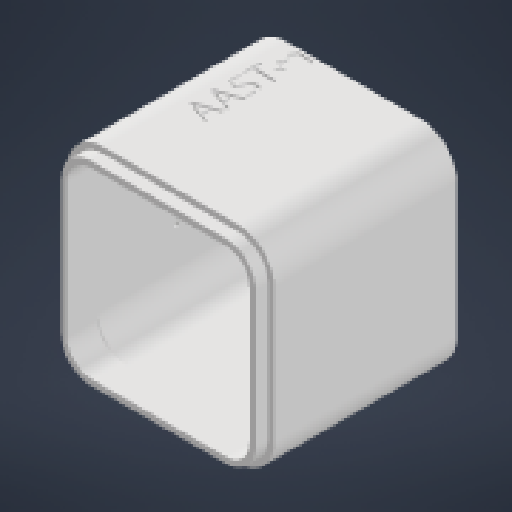
# Autodesk Inventor part: bottom case
Saved by Autodesk Inventor 2024 (Build 280153000, 153)
## iProperties
Created: 2023-06-18
Part Number: bottom case
Material: 일반
Document SubType Name: Modeling
Designer: 6gioc
Density: 1 g/cm^3
Appearance: 기본값
Author: 6gioc
Autodesk Inventor part; units mm, degrees
ref_plane "YZ Plane" through (0, 0, 0) normal (1, 0, 0) x (0, 1, 0)
ref_plane "XZ Plane" through (0, 0, 0) normal (0, 1, 0) x (-1, 0, 0)
ref_plane "XY Plane" through (0, 0, 0) normal (0, 0, 1) x (1, 0, 0)
sketch "스케치1" plane through (0, 0, 0) normal (0, 0, 1) x (1, 0, 0)
  line L0 (-30, 0) -> (-140, 0)
  line L1 (-170, -30) -> (-170, -140)
  line L2 (-140, -170) -> (-30, -170)
  line L3 (0, -140) -> (0, -30)
  arc A0 (-30, -170) -> (0, -140) centre (-30, -140) ccw
  arc A1 (-170, -140) -> (-140, -170) centre (-140, -140) ccw
  arc A2 (-140, 0) -> (-170, -30) centre (-140, -30) ccw
  arc A3 (0, -30) -> (-30, 0) centre (-30, -30) ccw
  point P0 (0, 0)
  point P1 (-170, -170)
  point P2 (-170, 0)
  point P3 (0, -170)
  dimension "d0" = 170
  dimension "d1" = 170
  dimension "d2" = 30
  dimension "d3" = 30
  dimension "d4" = 30
  constraints: 8 end point, 8 point on circle, 8 point on line, 8 tangent, 4 centre point, 2 parallel, 1 equal radius, 1 horizontal, 1 perpendicular
  measures "d0" distance of point (0, -170) point (-170, -170)
  measures "d1" distance of point (-170, -170) point (-170, 0)
  measures "d2" radius of A0
  measures "d3" radius of A1
  measures "d4" radius of A3
extrude "돌출1" add sketch "스케치1" along normal blind 150
shell "쉘1" thickness 5 removed faces 1 at (-66.6667, -113.3333, 150)
sketch "스케치2" plane through (0, 0, 150) normal (0, 0, 1) x (1, 0, 0)
  line L0 (-30, 0) -> (-140, 0)
  line L1 (-170, -30) -> (-170, -140)
  line L2 (-140, -170) -> (-30, -170)
  line L3 (0, -140) -> (0, -30)
  arc A0 (-30, -170) -> (0, -140) centre (-30, -140) ccw
  arc A1 (0, -30) -> (-30, 0) centre (-30, -30) ccw
  arc A2 (-140, 0) -> (-170, -30) centre (-140, -30) ccw
  arc A3 (-170, -140) -> (-140, -170) centre (-140, -140) ccw
  line L4 (-160, -30) -> (-160, -140)
  arc A4 (-160, -140) -> (-140, -160) centre (-140, -140) ccw
  line L5 (-140, -160) -> (-30, -160)
  arc A5 (-30, -160) -> (-10, -140) centre (-30, -140) ccw
  line L6 (-10, -140) -> (-10, -30)
  arc A6 (-10, -30) -> (-30, -10) centre (-30, -30) ccw
  line L7 (-30, -10) -> (-140, -10)
  arc A7 (-140, -10) -> (-160, -30) centre (-140, -30) ccw
  line L8 (-5, -140) -> (-5, -30)
  arc A8 (-5, -30) -> (-30, -5) centre (-30, -30) ccw
  line L9 (-30, -5) -> (-140, -5)
  arc A9 (-140, -5) -> (-165, -30) centre (-140, -30) ccw
  line L10 (-165, -30) -> (-165, -140)
  arc A10 (-165, -140) -> (-140, -165) centre (-140, -140) ccw
  line L11 (-140, -165) -> (-30, -165)
  arc A11 (-30, -165) -> (-5, -140) centre (-30, -140) ccw
  point P0 (0, 0)
  point P1 (-170, -170)
  point P2 (-170, 0)
  point P3 (0, -170)
  dimension "d8" = 170
  dimension "d9" = 170
  dimension "d10" = 30
  dimension "d11" = 10
  dimension "d17" = 5
  constraints: 24 end point, 24 point on circle, 12 centre point, 8 point on line, 8 tangent, 6 parallel, 3 equal radius, 3 perpendicular, 1 horizontal, 14 other
  measures "d8" distance of point (0, -170) point (-170, -170)
  measures "d9" distance of point (-170, -170) point (-170, 0)
  measures "d10" radius of A0
  measures "d11" radial gap between concentric circles of A2 A7
  measures "d17" radial gap between concentric circles of A0 A11
extrude "돌출2" add sketch "스케치2" against normal blind 20 contours A1 L3 A0 L2 A3 L1 A2 L0 | A11 L11 A10 L10 A9 L9 A8 L8
chamfer "모따기1" distance 5 angle 45 8 edges at (-85, -160, 130) (-15.8579, -154.1421, 130) (-10, -85, 130) (-15.8579, -15.8579, 130) (-85, -10, 130) (-154.1421, -15.8579, 130) (-160, -85, 130) (-154.1421, -154.1421, 130)
extrude "돌출3" add sketch "스케치2" along normal blind 10 contours A11 L11 A10 L10 A9 L9 A8 L8
sketch "스케치3" plane through (-140, 0, 0) normal (0, 1, 0) x (1, 0, 0)
  line L0 (23.785, -91.5699) -> (3.785, -84.2336)
  line L1 (3.785, -84.2336) -> (3.785, -81.9279)
  line L2 (3.785, -81.9279) -> (23.785, -74.6266)
  line L3 (23.785, -74.6266) -> (23.785, -77.107)
  line L4 (23.785, -77.107) -> (17.9509, -79.2205)
  line L5 (17.9509, -79.2205) -> (17.9509, -87.238)
  line L6 (17.9509, -87.238) -> (23.785, -89.2991)
  line L7 (23.785, -89.2991) -> (23.785, -91.5699)
  line L8 (6.9465, -83.2729) -> (15.9422, -86.5568)
  line L9 (15.9422, -86.5568) -> (15.9422, -79.9716)
  line L10 (15.9422, -79.9716) -> (6.9465, -83.2205)
  line L11 (6.9465, -83.2205) -> (6.9465, -83.2729)
  line L12 (23.785, -73.5262) -> (3.785, -66.1899)
  line L13 (3.785, -66.1899) -> (3.785, -63.8843)
  line L14 (3.785, -63.8843) -> (23.785, -56.583)
  line L15 (23.785, -56.583) -> (23.785, -59.0633)
  line L16 (23.785, -59.0633) -> (17.9509, -61.1768)
  line L17 (17.9509, -61.1768) -> (17.9509, -69.1943)
  line L18 (17.9509, -69.1943) -> (23.785, -71.2555)
  line L19 (23.785, -71.2555) -> (23.785, -73.5262)
  line L20 (6.9465, -65.2292) -> (15.9422, -68.5131)
  line L21 (15.9422, -68.5131) -> (15.9422, -61.9279)
  line L22 (15.9422, -61.9279) -> (6.9465, -65.1768)
  line L23 (6.9465, -65.1768) -> (6.9465, -65.2292)
  spline S0 degree 2 poles (24.1518, -49.1768) (24.1518, -52.4607) (22.8068, -54.8712) knots 0 0 0 1 1 1
  line L24 (22.8068, -54.8712) -> (20.8155, -54.8712)
  spline S1 degree 2 poles (20.8155, -54.8712) (22.1256, -52.321) (22.1256, -49.2817) knots 0 0 0 1 1 1
  spline S2 degree 2 poles (22.1256, -49.2817) (22.1256, -47.0284) (20.2042, -44.8624) (18.5098, -44.8624) knots 0 0 0 1 2 2 2
  spline S3 degree 2 poles (18.5098, -44.8624) (17.0251, -44.8624) (15.4356, -46.3821) (14.8417, -48.2511) knots 0 0 0 1 2 2 2
  line L25 (14.8417, -48.2511) -> (14.1605, -50.1899)
  spline S4 degree 2 poles (14.1605, -50.1899) (13.4094, -52.4083) (10.9465, -54.5742) (8.7631, -54.5742) knots 0 0 0 1 2 2 2
  spline S5 degree 2 poles (8.7631, -54.5742) (6.3526, -54.5742) (3.4531, -51.3952) (3.4531, -48.3559) knots 0 0 0 1 2 2 2
  spline S6 degree 2 poles (3.4531, -48.3559) (3.4531, -45.7533) (4.5535, -43.4825) knots 0 0 0 1 1 1
  line L26 (4.5535, -43.4825) -> (6.5622, -43.4825)
  spline S7 degree 2 poles (6.5622, -43.4825) (5.4443, -45.8755) (5.4443, -48.4432) knots 0 0 0 1 1 1
  spline S8 degree 2 poles (5.4443, -48.4432) (5.4443, -50.2598) (7.1212, -52.2511) (9.9858, -52.2511) (11.4705, -50.976) (12.0644, -49.2817) knots 0 0 0 1 2 3 4 4 4
  line L27 (12.0644, -49.2817) -> (12.6932, -47.3079)
  spline S9 degree 2 poles (12.6932, -47.3079) (13.5317, -44.8275) (15.9771, -42.4694) (18.3352, -42.4694) knots 0 0 0 1 2 2 2
  spline S10 degree 2 poles (18.3352, -42.4694) (21.0426, -42.4694) (24.1518, -45.7882) (24.1518, -49.1768) knots 0 0 0 1 2 2 2
  line L28 (23.785, -34.0677) -> (5.7762, -34.0677)
  line L29 (5.7762, -34.0677) -> (5.7762, -40.1812)
  line L30 (5.7762, -40.1812) -> (3.785, -40.1812)
  line L31 (3.785, -40.1812) -> (3.785, -25.631)
  line L32 (3.785, -25.631) -> (5.7762, -25.631)
  line L33 (5.7762, -25.631) -> (5.7762, -31.7445)
  line L34 (5.7762, -31.7445) -> (23.785, -31.7445)
  line L35 (23.785, -31.7445) -> (23.785, -34.0677)
  spline S11 degree 2 poles (9.9173, -17.3252) (11.1446, -16.9103) (12.5448, -14.4038) (12.5448, -13.1592) knots 0 0 0 1 2 2 2
  spline S12 degree 2 poles (12.5448, -13.1592) (12.5448, -11.6208) (10.9199, -8.9587) (9.416, -8.5438) knots 0 0 0 1 2 2 2
  spline S13 degree 2 poles (9.416, -8.5438) (9.8481, -6.7979) (11.8706, -3.7037) (12.804, -3.0469) knots 0 0 0 1 2 2 2
  spline S14 degree 2 poles (12.804, -3.0469) (13.8585, -2.3208) (15.2068, -2.3208) knots 0 0 0 1 1 1
  spline S15 degree 2 poles (15.2068, -2.3208) (16.123, -2.3208) (17.2811, -2.7703) knots 0 0 0 1 1 1
  spline S16 degree 2 poles (17.2811, -2.7703) (18.1973, -3.2197) (18.8369, -3.2197) knots 0 0 0 1 1 1
  spline S17 degree 2 poles (18.8369, -3.2197) (19.3036, -3.2197) (20.8594, -2.5801) knots 0 0 0 1 1 1
  spline S18 degree 2 poles (20.8594, -2.5801) (21.8447, -2.2863) (22.3114, -2.2863) knots 0 0 0 1 1 1
  spline S19 degree 2 poles (22.3114, -2.2863) (23.6943, -2.2863) (25.1117, -3.4617) knots 0 0 0 1 1 1
  spline S20 degree 2 poles (25.1117, -3.4617) (27.0651, -5.2422) (29.2258, -10.3243) (29.2258, -13.1074) knots 0 0 0 1 2 2 2
  spline S21 degree 2 poles (29.2258, -13.1074) (29.2258, -16.0114) (25.8378, -20.4367) (23.2103, -20.4367) knots 0 0 0 1 2 2 2
  spline S22 degree 2 poles (23.2103, -20.4367) (21.7755, -20.4367) (20.5482, -19.8144) knots 0 0 0 1 1 1
  spline S23 degree 2 poles (20.5482, -19.8144) (19.7185, -19.2958) (18.8715, -19.2958) knots 0 0 0 1 1 1
  spline S24 degree 2 poles (18.8715, -19.2958) (18.059, -19.2958) (17.2811, -19.6242) knots 0 0 0 1 1 1
  spline S25 degree 2 poles (17.2811, -19.6242) (15.2241, -20.4367) (14.4981, -20.4367) knots 0 0 0 1 1 1
  spline S26 degree 2 poles (14.4981, -20.4367) (12.5102, -20.4367) (11.0063, -19.0883) knots 0 0 0 1 1 1
  spline S27 degree 2 poles (11.0063, -19.0883) (10.384, -18.466) (9.9173, -17.3252) knots 0 0 0 1 1 1
  spline S28 degree 2 poles (19.7531, -19.6934) (19.7531, -21.8023) (18.3183, -23.5654) knots 0 0 0 1 1 1
  spline S29 degree 2 poles (18.3183, -23.5654) (16.97, -25.0348) (14.5672, -25.3805) knots 0 0 0 1 1 1
  spline S30 degree 2 poles (14.5672, -25.3805) (14.5672, -22.9604) (15.9328, -21.3528) knots 0 0 0 1 1 1
  spline S31 degree 2 poles (15.9328, -21.3528) (17.454, -19.6934) (19.7531, -19.6934) knots 0 0 0 1 1 1
  point P0 (140, 0)
  point P1 (3.4531, -92.1288)
  dimension "d0" = 170
  dimension "d1" = 170
  dimension "d2" = 30
  dimension "d3" = 30
  dimension "d4" = 30
  constraints: 1 other
extrude "돌출4" cut sketch "스케치3" against normal blind 2
sketch "스케치4" plane through (-140, -170, 0) normal (0, -1, 0) x (1, 0, 0)
  line L0 (-0.2518, 6.8609) -> (110.1783, 6.8609) construction
  line L1 (110.1783, 6.8609) -> (110.1783, 29.5331) construction
  line L2 (110.1783, 29.5331) -> (-0.2518, 29.5331) construction
  line L3 (-0.2518, 29.5331) -> (-0.2518, 6.8609) construction
  line L4 (6.2831, 27.3688) -> (5.0902, 27.3688)
  line L5 (5.0902, 27.3688) -> (1.5505, 34.2667)
  line L6 (1.5505, 34.2667) -> (1.5505, 27.3688)
  line L7 (1.5505, 27.3688) -> (0.5586, 27.3688)
  line L8 (0.5586, 27.3688) -> (0.5586, 35.3688)
  line L9 (0.5586, 35.3688) -> (2.0692, 35.3688)
  line L10 (2.0692, 35.3688) -> (5.2912, 29.0349)
  line L11 (5.2912, 29.0349) -> (5.2912, 35.3688)
  line L12 (5.2912, 35.3688) -> (6.2831, 35.3688)
  line L13 (6.2831, 35.3688) -> (6.2831, 27.3688)
  spline S0 degree 2 poles (13.5635, 34.4547) (14.0173, 33.9231) (14.523, 32.3672) (14.523, 31.3688) knots 0 0 0 1 2 2 2
  spline S1 degree 2 poles (14.523, 31.3688) (14.523, 30.3964) (14.0303, 28.821) (13.5635, 28.2894) knots 0 0 0 1 2 2 2
  spline S2 degree 2 poles (13.5635, 28.2894) (13.0708, 27.7319) (11.7677, 27.2002) (10.9833, 27.2002) knots 0 0 0 1 2 2 2
  spline S3 degree 2 poles (10.9833, 27.2002) (10.1729, 27.2002) (8.8763, 27.7513) (8.403, 28.2894) knots 0 0 0 1 2 2 2
  spline S4 degree 2 poles (8.403, 28.2894) (7.9427, 28.821) (7.45, 30.3834) (7.45, 31.3688) knots 0 0 0 1 2 2 2
  spline S5 degree 2 poles (7.45, 31.3688) (7.45, 32.3737) (7.9492, 33.9037) (8.4095, 34.4547) knots 0 0 0 1 2 2 2
  spline S6 degree 2 poles (8.4095, 34.4547) (8.8763, 34.9863) (10.1794, 35.5374) (10.9833, 35.5374) knots 0 0 0 1 2 2 2
  spline S7 degree 2 poles (10.9833, 35.5374) (11.8001, 35.5374) (13.1097, 34.9669) (13.5635, 34.4547) knots 0 0 0 1 2 2 2
  spline S8 degree 2 poles (13.4144, 31.3688) (13.4144, 32.1597) (13.0708, 33.385) (12.7596, 33.787) knots 0 0 0 1 2 2 2
  spline S9 degree 2 poles (12.7596, 33.787) (12.4419, 34.2019) (11.5473, 34.6168) (10.9897, 34.6168) knots 0 0 0 1 2 2 2
  spline S10 degree 2 poles (10.9897, 34.6168) (10.4128, 34.6168) (9.544, 34.2148) (9.2134, 33.787) knots 0 0 0 1 2 2 2
  spline S11 degree 2 poles (9.2134, 33.787) (8.8957, 33.3785) (8.5586, 32.1468) (8.5586, 31.3688) knots 0 0 0 1 2 2 2
  spline S12 degree 2 poles (8.5586, 31.3688) (8.5586, 29.7934) (9.8811, 28.1208) (10.9897, 28.1208) knots 0 0 0 1 2 2 2
  spline S13 degree 2 poles (10.9897, 28.1208) (12.0983, 28.1208) (13.4144, 29.7934) (13.4144, 31.3688) knots 0 0 0 1 2 2 2
  line L14 (17.557, 27.3688) -> (17.557, 34.4223)
  line L15 (17.557, 34.4223) -> (14.873, 34.4223)
  line L16 (14.873, 34.4223) -> (14.873, 35.3688)
  line L17 (14.873, 35.3688) -> (21.3042, 35.3688)
  line L18 (21.3042, 35.3688) -> (21.3042, 34.4223)
  line L19 (21.3042, 34.4223) -> (18.6202, 34.4223)
  line L20 (18.6202, 34.4223) -> (18.6202, 27.3688)
  line L21 (18.6202, 27.3688) -> (17.557, 27.3688)
  line L22 (30.335, 34.4223) -> (26.6137, 34.4223)
  line L23 (26.6137, 34.4223) -> (26.6137, 32.1662)
  line L24 (26.6137, 32.1662) -> (30.1794, 32.1662)
  line L25 (30.1794, 32.1662) -> (30.1794, 31.2197)
  line L26 (30.1794, 31.2197) -> (26.6137, 31.2197)
  line L27 (26.6137, 31.2197) -> (26.6137, 27.3688)
  line L28 (26.6137, 27.3688) -> (25.5505, 27.3688)
  line L29 (25.5505, 27.3688) -> (25.5505, 35.3688)
  line L30 (25.5505, 35.3688) -> (30.335, 35.3688)
  line L31 (30.335, 35.3688) -> (30.335, 34.4223)
  spline S14 degree 2 poles (36.9476, 34.4547) (37.4014, 33.9231) (37.9071, 32.3672) (37.9071, 31.3688) knots 0 0 0 1 2 2 2
  spline S15 degree 2 poles (37.9071, 31.3688) (37.9071, 30.3964) (37.4144, 28.821) (36.9476, 28.2894) knots 0 0 0 1 2 2 2
  spline S16 degree 2 poles (36.9476, 28.2894) (36.4549, 27.7319) (35.1518, 27.2002) (34.3674, 27.2002) knots 0 0 0 1 2 2 2
  spline S17 degree 2 poles (34.3674, 27.2002) (33.557, 27.2002) (32.2604, 27.7513) (31.7871, 28.2894) knots 0 0 0 1 2 2 2
  spline S18 degree 2 poles (31.7871, 28.2894) (31.3269, 28.821) (30.8341, 30.3834) (30.8341, 31.3688) knots 0 0 0 1 2 2 2
  spline S19 degree 2 poles (30.8341, 31.3688) (30.8341, 32.3737) (31.3333, 33.9037) (31.7936, 34.4547) knots 0 0 0 1 2 2 2
  spline S20 degree 2 poles (31.7936, 34.4547) (32.2604, 34.9863) (33.5635, 35.5374) (34.3674, 35.5374) knots 0 0 0 1 2 2 2
  spline S21 degree 2 poles (34.3674, 35.5374) (35.1842, 35.5374) (36.4938, 34.9669) (36.9476, 34.4547) knots 0 0 0 1 2 2 2
  spline S22 degree 2 poles (36.7985, 31.3688) (36.7985, 32.1597) (36.4549, 33.385) (36.1437, 33.787) knots 0 0 0 1 2 2 2
  spline S23 degree 2 poles (36.1437, 33.787) (35.826, 34.2019) (34.9314, 34.6168) (34.3739, 34.6168) knots 0 0 0 1 2 2 2
  spline S24 degree 2 poles (34.3739, 34.6168) (33.7969, 34.6168) (32.9281, 34.2148) (32.5975, 33.787) knots 0 0 0 1 2 2 2
  spline S25 degree 2 poles (32.5975, 33.787) (32.2799, 33.3785) (31.9427, 32.1468) (31.9427, 31.3688) knots 0 0 0 1 2 2 2
  spline S26 degree 2 poles (31.9427, 31.3688) (31.9427, 29.7934) (33.2653, 28.1208) (34.3739, 28.1208) knots 0 0 0 1 2 2 2
  spline S27 degree 2 poles (34.3739, 28.1208) (35.4824, 28.1208) (36.7985, 29.7934) (36.7985, 31.3688) knots 0 0 0 1 2 2 2
  line L32 (45.2653, 27.3688) -> (43.8844, 27.3688)
  line L33 (43.8844, 27.3688) -> (41.356, 30.552)
  line L34 (41.356, 30.552) -> (40.1372, 30.552)
  line L35 (40.1372, 30.552) -> (40.1372, 27.3688)
  line L36 (40.1372, 27.3688) -> (39.074, 27.3688)
  line L37 (39.074, 27.3688) -> (39.074, 35.3688)
  line L38 (39.074, 35.3688) -> (41.1356, 35.3688)
  spline S28 degree 2 poles (41.1356, 35.3688) (41.8228, 35.3688) (42.7499, 35.2197) (43.1713, 34.9474) knots 0 0 0 1 2 2 2
  spline S29 degree 2 poles (43.1713, 34.9474) (43.5927, 34.6751) (44.0789, 33.8259) (44.0789, 33.197) knots 0 0 0 1 2 2 2
  spline S30 degree 2 poles (44.0789, 33.197) (44.0789, 32.3218) (43.1842, 31.1354) (42.4192, 30.8502) knots 0 0 0 1 2 2 2
  line L39 (42.4192, 30.8502) -> (45.2653, 27.3688)
  spline S31 degree 2 poles (42.9703, 33.1127) (42.9703, 33.4628) (42.7239, 34.0009) (42.4646, 34.1759) knots 0 0 0 1 2 2 2
  spline S32 degree 2 poles (42.4646, 34.1759) (42.2377, 34.325) (41.6348, 34.4482) (41.194, 34.4482) knots 0 0 0 1 2 2 2
  line L40 (41.194, 34.4482) -> (40.1372, 34.4482)
  line L41 (40.1372, 34.4482) -> (40.1372, 31.4401)
  line L42 (40.1372, 31.4401) -> (41.0708, 31.4401)
  spline S33 degree 2 poles (41.0708, 31.4401) (41.5311, 31.4401) (42.2636, 31.6022) (42.5165, 31.855) knots 0 0 0 1 2 2 2
  spline S34 degree 2 poles (42.5165, 31.855) (42.7499, 32.0755) (42.9703, 32.6978) (42.9703, 33.1127) knots 0 0 0 1 2 2 2
  line L43 (7.4176, 14.197) -> (6.3544, 14.197)
  line L44 (6.3544, 14.197) -> (6.3544, 21.0884)
  line L45 (6.3544, 21.0884) -> (4.2669, 16.4012)
  line L46 (4.2669, 16.4012) -> (3.6186, 16.4012)
  line L47 (3.6186, 16.4012) -> (1.5505, 21.0884)
  line L48 (1.5505, 21.0884) -> (1.5505, 14.197)
  line L49 (1.5505, 14.197) -> (0.5586, 14.197)
  line L50 (0.5586, 14.197) -> (0.5586, 22.197)
  line L51 (0.5586, 22.197) -> (2.0108, 22.197)
  line L52 (2.0108, 22.197) -> (4.0076, 17.7432)
  line L53 (4.0076, 17.7432) -> (5.9395, 22.197)
  line L54 (5.9395, 22.197) -> (7.4176, 22.197)
  line L55 (7.4176, 22.197) -> (7.4176, 14.197)
  line L56 (11.826, 14.197) -> (8.7272, 14.197)
  line L57 (8.7272, 14.197) -> (8.7272, 15.0139)
  line L58 (8.7272, 15.0139) -> (9.745, 15.0139)
  line L59 (9.745, 15.0139) -> (9.745, 21.3802)
  line L60 (9.745, 21.3802) -> (8.7272, 21.3802)
  line L61 (8.7272, 21.3802) -> (8.7272, 22.197)
  line L62 (8.7272, 22.197) -> (11.826, 22.197)
  line L63 (11.826, 22.197) -> (11.826, 21.3802)
  line L64 (11.826, 21.3802) -> (10.8082, 21.3802)
  line L65 (10.8082, 21.3802) -> (10.8082, 15.0139)
  line L66 (10.8082, 15.0139) -> (11.826, 15.0139)
  line L67 (11.826, 15.0139) -> (11.826, 14.197)
  line L68 (17.7774, 14.197) -> (13.1421, 14.197)
  line L69 (13.1421, 14.197) -> (13.1421, 22.197)
  line L70 (13.1421, 22.197) -> (14.2053, 22.197)
  line L71 (14.2053, 22.197) -> (14.2053, 15.1435)
  line L72 (14.2053, 15.1435) -> (17.7774, 15.1435)
  line L73 (17.7774, 15.1435) -> (17.7774, 14.197)
  line L74 (21.4014, 14.197) -> (18.3025, 14.197)
  line L75 (18.3025, 14.197) -> (18.3025, 15.0139)
  line L76 (18.3025, 15.0139) -> (19.3204, 15.0139)
  line L77 (19.3204, 15.0139) -> (19.3204, 21.3802)
  line L78 (19.3204, 21.3802) -> (18.3025, 21.3802)
  line L79 (18.3025, 21.3802) -> (18.3025, 22.197)
  line L80 (18.3025, 22.197) -> (21.4014, 22.197)
  line L81 (21.4014, 22.197) -> (21.4014, 21.3802)
  line L82 (21.4014, 21.3802) -> (20.3836, 21.3802)
  line L83 (20.3836, 21.3802) -> (20.3836, 15.0139)
  line L84 (20.3836, 15.0139) -> (21.4014, 15.0139)
  line L85 (21.4014, 15.0139) -> (21.4014, 14.197)
  line L86 (24.5846, 14.197) -> (24.5846, 21.2505)
  line L87 (24.5846, 21.2505) -> (21.9006, 21.2505)
  line L88 (21.9006, 21.2505) -> (21.9006, 22.197)
  line L89 (21.9006, 22.197) -> (28.3317, 22.197)
  line L90 (28.3317, 22.197) -> (28.3317, 21.2505)
  line L91 (28.3317, 21.2505) -> (25.6478, 21.2505)
  line L92 (25.6478, 21.2505) -> (25.6478, 14.197)
  line L93 (25.6478, 14.197) -> (24.5846, 14.197)
  line L94 (28.2799, 14.197) -> (30.9768, 22.197)
  line L95 (30.9768, 22.197) -> (32.2863, 22.197)
  line L96 (32.2863, 22.197) -> (34.9833, 14.197)
  line L97 (34.9833, 14.197) -> (33.8617, 14.197)
  line L98 (33.8617, 14.197) -> (33.1356, 16.4336)
  line L99 (33.1356, 16.4336) -> (30.0821, 16.4336)
  line L100 (30.0821, 16.4336) -> (29.356, 14.197)
  line L101 (29.356, 14.197) -> (28.2799, 14.197)
  line L102 (32.8439, 17.3413) -> (31.6056, 21.1079)
  line L103 (31.6056, 21.1079) -> (30.3739, 17.3413)
  line L104 (30.3739, 17.3413) -> (32.8439, 17.3413)
  line L105 (41.933, 14.197) -> (40.5521, 14.197)
  line L106 (40.5521, 14.197) -> (38.0238, 17.3802)
  line L107 (38.0238, 17.3802) -> (36.805, 17.3802)
  line L108 (36.805, 17.3802) -> (36.805, 14.197)
  line L109 (36.805, 14.197) -> (35.7418, 14.197)
  line L110 (35.7418, 14.197) -> (35.7418, 22.197)
  line L111 (35.7418, 22.197) -> (37.8034, 22.197)
  spline S35 degree 2 poles (37.8034, 22.197) (38.4905, 22.197) (39.4176, 22.0479) (39.839, 21.7756) knots 0 0 0 1 2 2 2
  spline S36 degree 2 poles (39.839, 21.7756) (40.2604, 21.5033) (40.7466, 20.6541) (40.7466, 20.0252) knots 0 0 0 1 2 2 2
  spline S37 degree 2 poles (40.7466, 20.0252) (40.7466, 19.15) (39.852, 17.9636) (39.087, 17.6784) knots 0 0 0 1 2 2 2
  line L112 (39.087, 17.6784) -> (41.933, 14.197)
  spline S38 degree 2 poles (39.638, 19.9409) (39.638, 20.291) (39.3917, 20.8291) (39.1324, 21.0041) knots 0 0 0 1 2 2 2
  spline S39 degree 2 poles (39.1324, 21.0041) (38.9055, 21.1533) (38.3025, 21.2764) (37.8617, 21.2764) knots 0 0 0 1 2 2 2
  line L113 (37.8617, 21.2764) -> (36.805, 21.2764)
  line L114 (36.805, 21.2764) -> (36.805, 18.2683)
  line L115 (36.805, 18.2683) -> (37.7385, 18.2683)
  spline S40 degree 2 poles (37.7385, 18.2683) (38.1988, 18.2683) (38.9314, 18.4304) (39.1842, 18.6832) knots 0 0 0 1 2 2 2
  spline S41 degree 2 poles (39.1842, 18.6832) (39.4176, 18.9037) (39.638, 19.526) (39.638, 19.9409) knots 0 0 0 1 2 2 2
  line L116 (48.1696, 22.197) -> (45.4662, 17.7367)
  line L117 (45.4662, 17.7367) -> (45.4662, 14.197)
  line L118 (45.4662, 14.197) -> (44.403, 14.197)
  line L119 (44.403, 14.197) -> (44.403, 17.6265)
  line L120 (44.403, 17.6265) -> (41.6996, 22.197)
  line L121 (41.6996, 22.197) -> (42.8795, 22.197)
  line L122 (42.8795, 22.197) -> (44.9411, 18.6768)
  line L123 (44.9411, 18.6768) -> (47.0416, 22.197)
  line L124 (47.0416, 22.197) -> (48.1696, 22.197)
  spline S42 degree 2 poles (5.6153, 6.6136) (5.6153, 6.0949) (5.2458, 5.1614) (4.9152, 4.8372) knots 0 0 0 1 2 2 2
  spline S43 degree 2 poles (4.9152, 4.8372) (4.5003, 4.4288) (3.3787, 4.0074) (2.523, 4.0074) knots 0 0 0 1 2 2 2
  line L125 (2.523, 4.0074) -> (1.6218, 4.0074)
  line L126 (1.6218, 4.0074) -> (1.6218, 1.0252)
  line L127 (1.6218, 1.0252) -> (0.5586, 1.0252)
  line L128 (0.5586, 1.0252) -> (0.5586, 9.0252)
  line L129 (0.5586, 9.0252) -> (2.5683, 9.0252)
  spline S44 degree 2 poles (2.5683, 9.0252) (3.2815, 9.0252) (4.2799, 8.7918) (4.6623, 8.526) knots 0 0 0 1 2 2 2
  spline S45 degree 2 poles (4.6623, 8.526) (5.1097, 8.2213) (5.6153, 7.2813) (5.6153, 6.6136) knots 0 0 0 1 2 2 2
  spline S46 degree 2 poles (4.5068, 6.5811) (4.5068, 6.9961) (4.2215, 7.6055) (3.9298, 7.7999) knots 0 0 0 1 2 2 2
  spline S47 degree 2 poles (3.9298, 7.7999) (3.6769, 7.9685) (3.0027, 8.1046) (2.5035, 8.1046) knots 0 0 0 1 2 2 2
  line L130 (2.5035, 8.1046) -> (1.6218, 8.1046)
  line L131 (1.6218, 8.1046) -> (1.6218, 4.915)
  line L132 (1.6218, 4.915) -> (2.3479, 4.915)
  spline S48 degree 2 poles (2.3479, 4.915) (2.9962, 4.915) (3.7936, 5.1225) (4.0529, 5.3948) knots 0 0 0 1 2 2 2
  spline S49 degree 2 poles (4.0529, 5.3948) (4.2928, 5.6346) (4.5068, 6.1986) (4.5068, 6.5811) knots 0 0 0 1 2 2 2
  line L133 (6.6267, 1.0252) -> (6.6267, 9.0252)
  line L134 (6.6267, 9.0252) -> (11.6316, 9.0252)
  line L135 (11.6316, 9.0252) -> (11.6316, 8.0787)
  line L136 (11.6316, 8.0787) -> (7.6899, 8.0787)
  line L137 (7.6899, 8.0787) -> (7.6899, 5.8875)
  line L138 (7.6899, 5.8875) -> (11.3658, 5.8875)
  line L139 (11.3658, 5.8875) -> (11.3658, 4.941)
  line L140 (11.3658, 4.941) -> (7.6899, 4.941)
  line L141 (7.6899, 4.941) -> (7.6899, 1.9717)
  line L142 (7.6899, 1.9717) -> (11.6316, 1.9717)
  line L143 (11.6316, 1.9717) -> (11.6316, 1.0252)
  line L144 (11.6316, 1.0252) -> (6.6267, 1.0252)
  line L145 (18.9897, 1.0252) -> (17.6089, 1.0252)
  line L146 (17.6089, 1.0252) -> (15.0805, 4.2084)
  line L147 (15.0805, 4.2084) -> (13.8617, 4.2084)
  line L148 (13.8617, 4.2084) -> (13.8617, 1.0252)
  line L149 (13.8617, 1.0252) -> (12.7985, 1.0252)
  line L150 (12.7985, 1.0252) -> (12.7985, 9.0252)
  line L151 (12.7985, 9.0252) -> (14.8601, 9.0252)
  spline S50 degree 2 poles (14.8601, 9.0252) (15.5473, 9.0252) (16.4743, 8.8761) (16.8957, 8.6038) knots 0 0 0 1 2 2 2
  spline S51 degree 2 poles (16.8957, 8.6038) (17.3171, 8.3316) (17.8034, 7.4823) (17.8034, 6.8534) knots 0 0 0 1 2 2 2
  spline S52 degree 2 poles (17.8034, 6.8534) (17.8034, 5.9782) (16.9087, 4.7918) (16.1437, 4.5066) knots 0 0 0 1 2 2 2
  line L152 (16.1437, 4.5066) -> (18.9897, 1.0252)
  spline S53 degree 2 poles (16.6948, 6.7692) (16.6948, 7.1192) (16.4484, 7.6573) (16.1891, 7.8324) knots 0 0 0 1 2 2 2
  spline S54 degree 2 poles (16.1891, 7.8324) (15.9622, 7.9815) (15.3593, 8.1046) (14.9184, 8.1046) knots 0 0 0 1 2 2 2
  line L153 (14.9184, 8.1046) -> (13.8617, 8.1046)
  line L154 (13.8617, 8.1046) -> (13.8617, 5.0965)
  line L155 (13.8617, 5.0965) -> (14.7952, 5.0965)
  spline S55 degree 2 poles (14.7952, 5.0965) (15.2555, 5.0965) (15.9881, 5.2586) (16.241, 5.5115) knots 0 0 0 1 2 2 2
  spline S56 degree 2 poles (16.241, 5.5115) (16.4743, 5.7319) (16.6948, 6.3542) (16.6948, 6.7692) knots 0 0 0 1 2 2 2
  spline S57 degree 2 poles (24.6818, 6.6136) (24.6818, 6.0949) (24.3123, 5.1614) (23.9816, 4.8372) knots 0 0 0 1 2 2 2
  spline S58 degree 2 poles (23.9816, 4.8372) (23.5667, 4.4288) (22.4452, 4.0074) (21.5894, 4.0074) knots 0 0 0 1 2 2 2
  line L156 (21.5894, 4.0074) -> (20.6883, 4.0074)
  line L157 (20.6883, 4.0074) -> (20.6883, 1.0252)
  line L158 (20.6883, 1.0252) -> (19.6251, 1.0252)
  line L159 (19.6251, 1.0252) -> (19.6251, 9.0252)
  line L160 (19.6251, 9.0252) -> (21.6348, 9.0252)
  spline S59 degree 2 poles (21.6348, 9.0252) (22.3479, 9.0252) (23.3463, 8.7918) (23.7288, 8.526) knots 0 0 0 1 2 2 2
  spline S60 degree 2 poles (23.7288, 8.526) (24.1761, 8.2213) (24.6818, 7.2813) (24.6818, 6.6136) knots 0 0 0 1 2 2 2
  spline S61 degree 2 poles (23.5732, 6.5811) (23.5732, 6.9961) (23.288, 7.6055) (22.9962, 7.7999) knots 0 0 0 1 2 2 2
  spline S62 degree 2 poles (22.9962, 7.7999) (22.7434, 7.9685) (22.0692, 8.1046) (21.57, 8.1046) knots 0 0 0 1 2 2 2
  line L161 (21.57, 8.1046) -> (20.6883, 8.1046)
  line L162 (20.6883, 8.1046) -> (20.6883, 4.915)
  line L163 (20.6883, 4.915) -> (21.4144, 4.915)
  spline S63 degree 2 poles (21.4144, 4.915) (22.0627, 4.915) (22.8601, 5.1225) (23.1194, 5.3948) knots 0 0 0 1 2 2 2
  spline S64 degree 2 poles (23.1194, 5.3948) (23.3593, 5.6346) (23.5732, 6.1986) (23.5732, 6.5811) knots 0 0 0 1 2 2 2
  spline S65 degree 2 poles (31.3528, 8.1111) (31.8066, 7.5795) (32.3123, 6.0236) (32.3123, 5.0252) knots 0 0 0 1 2 2 2
  spline S66 degree 2 poles (32.3123, 5.0252) (32.3123, 4.0528) (31.8196, 2.4774) (31.3528, 1.9458) knots 0 0 0 1 2 2 2
  spline S67 degree 2 poles (31.3528, 1.9458) (30.8601, 1.3883) (29.557, 0.8567) (28.7726, 0.8567) knots 0 0 0 1 2 2 2
  spline S68 degree 2 poles (28.7726, 0.8567) (27.9622, 0.8567) (26.6656, 1.4077) (26.1923, 1.9458) knots 0 0 0 1 2 2 2
  spline S69 degree 2 poles (26.1923, 1.9458) (25.732, 2.4774) (25.2393, 4.0398) (25.2393, 5.0252) knots 0 0 0 1 2 2 2
  spline S70 degree 2 poles (25.2393, 5.0252) (25.2393, 6.0301) (25.7385, 7.5601) (26.1988, 8.1111) knots 0 0 0 1 2 2 2
  spline S71 degree 2 poles (26.1988, 8.1111) (26.6656, 8.6427) (27.9687, 9.1938) (28.7726, 9.1938) knots 0 0 0 1 2 2 2
  spline S72 degree 2 poles (28.7726, 9.1938) (29.5894, 9.1938) (30.899, 8.6233) (31.3528, 8.1111) knots 0 0 0 1 2 2 2
  spline S73 degree 2 poles (31.2037, 5.0252) (31.2037, 5.8162) (30.8601, 7.0414) (30.5489, 7.4434) knots 0 0 0 1 2 2 2
  spline S74 degree 2 poles (30.5489, 7.4434) (30.2312, 7.8583) (29.3366, 8.2732) (28.779, 8.2732) knots 0 0 0 1 2 2 2
  spline S75 degree 2 poles (28.779, 8.2732) (28.2021, 8.2732) (27.3333, 7.8713) (27.0027, 7.4434) knots 0 0 0 1 2 2 2
  spline S76 degree 2 poles (27.0027, 7.4434) (26.685, 7.035) (26.3479, 5.8032) (26.3479, 5.0252) knots 0 0 0 1 2 2 2
  spline S77 degree 2 poles (26.3479, 5.0252) (26.3479, 3.4499) (27.6705, 1.7773) (28.779, 1.7773) knots 0 0 0 1 2 2 2
  spline S78 degree 2 poles (28.779, 1.7773) (29.8876, 1.7773) (31.2037, 3.4499) (31.2037, 5.0252) knots 0 0 0 1 2 2 2
  spline S79 degree 2 poles (35.7093, 0.8826) (34.8406, 0.8826) (33.6218, 1.2457) (33.0837, 1.505) knots 0 0 0 1 2 2 2
  line L164 (33.0837, 1.505) -> (33.0837, 2.8405)
  line L165 (33.0837, 2.8405) -> (33.1615, 2.8405)
  spline S80 degree 2 poles (33.1615, 2.8405) (33.6867, 2.3478) (35.0157, 1.8032) (35.6316, 1.8032) knots 0 0 0 1 2 2 2
  spline S81 degree 2 poles (35.6316, 1.8032) (36.5132, 1.8032) (37.4144, 2.5358) (37.4144, 3.1387) knots 0 0 0 1 2 2 2
  spline S82 degree 2 poles (37.4144, 3.1387) (37.4144, 3.6184) (36.9411, 4.2149) (36.429, 4.364) knots 0 0 0 1 2 2 2
  spline S83 degree 2 poles (36.429, 4.364) (36.0594, 4.4677) (35.4435, 4.6103) (34.9833, 4.727) knots 0 0 0 1 2 2 2
  spline S84 degree 2 poles (34.9833, 4.727) (34.5683, 4.8372) (33.9136, 5.1679) (33.6607, 5.4337) knots 0 0 0 1 2 2 2
  spline S85 degree 2 poles (33.6607, 5.4337) (33.4144, 5.6995) (33.1421, 6.4126) (33.1421, 6.8794) knots 0 0 0 1 2 2 2
  spline S86 degree 2 poles (33.1421, 6.8794) (33.1421, 7.8518) (34.6591, 9.1679) (35.8325, 9.1679) knots 0 0 0 1 2 2 2
  spline S87 degree 2 poles (35.8325, 9.1679) (36.5068, 9.1679) (37.6996, 8.9021) (38.2118, 8.6492) knots 0 0 0 1 2 2 2
  line L166 (38.2118, 8.6492) -> (38.2118, 7.3786)
  line L167 (38.2118, 7.3786) -> (38.134, 7.3786)
  spline S88 degree 2 poles (38.134, 7.3786) (37.7515, 7.7286) (36.5586, 8.2473) (35.9038, 8.2473) knots 0 0 0 1 2 2 2
  spline S89 degree 2 poles (35.9038, 8.2473) (35.1648, 8.2473) (34.2507, 7.5536) (34.2507, 6.9896) knots 0 0 0 1 2 2 2
  spline S90 degree 2 poles (34.2507, 6.9896) (34.2507, 6.4839) (34.7888, 5.881) (35.2944, 5.7448) knots 0 0 0 1 2 2 2
  spline S91 degree 2 poles (35.2944, 5.7448) (35.6316, 5.6541) (36.6105, 5.4207) (36.9346, 5.3234) knots 0 0 0 1 2 2 2
  spline S92 degree 2 poles (36.9346, 5.3234) (37.758, 5.0706) (38.523, 4.0528) (38.523, 3.3072) knots 0 0 0 1 2 2 2
  spline S93 degree 2 poles (38.523, 3.3072) (38.523, 2.834) (38.1405, 1.9264) (37.7969, 1.6087) knots 0 0 0 1 2 2 2
  spline S94 degree 2 poles (37.7969, 1.6087) (37.4144, 1.2586) (36.4419, 0.8826) (35.7093, 0.8826) knots 0 0 0 1 2 2 2
  line L168 (39.6056, 1.0252) -> (39.6056, 9.0252)
  line L169 (39.6056, 9.0252) -> (44.6105, 9.0252)
  line L170 (44.6105, 9.0252) -> (44.6105, 8.0787)
  line L171 (44.6105, 8.0787) -> (40.6688, 8.0787)
  line L172 (40.6688, 8.0787) -> (40.6688, 5.8875)
  line L173 (40.6688, 5.8875) -> (44.3447, 5.8875)
  line L174 (44.3447, 5.8875) -> (44.3447, 4.941)
  line L175 (44.3447, 4.941) -> (40.6688, 4.941)
  line L176 (40.6688, 4.941) -> (40.6688, 1.9717)
  line L177 (40.6688, 1.9717) -> (44.6105, 1.9717)
  line L178 (44.6105, 1.9717) -> (44.6105, 1.0252)
  line L179 (44.6105, 1.0252) -> (39.6056, 1.0252)
  point P0 (140, 0)
  dimension "d0" = 170
  dimension "d1" = 170
  dimension "d2" = 30
  dimension "d3" = 30
  dimension "d4" = 30
  constraints: 2 other
extrude "돌출5" cut sketch "스케치4" against normal blind 2
sketch "스케치6" plane through (-170, -140, 0) normal (-1, 0, 0) x (0, 0, 1)
  line L0 (70, 85) -> (10, 85)
  line L1 (10, 85) -> (10, 25)
  line L2 (10, 25) -> (70, 25)
  line L3 (70, 25) -> (70, 85)
  line L4 (0, 0) -> (150, 0) projected
  line L5 (0, 110) -> (150, 110) projected
  line L6 (0, 110) -> (0, 0) projected
  circle A0 centre (65, 80) radius 2.15
  circle A1 centre (65, 30) radius 2.15
  circle A2 centre (15, 30) radius 2.15
  circle A3 centre (15, 80) radius 2.15
  circle A4 centre (40, 55) radius 27.5
  point P0 (0, 140)
  point P1 (40, 85)
  dimension "d44" = 60
  dimension "d45" = 60
  dimension "d46" = 110
  dimension "d47" = 25
  dimension "d50" = 10
  dimension "d51" = 4.3
  dimension "d52" = 4.3
  dimension "d53" = 4.3
  dimension "d54" = 4.3
  dimension "d55" = 50
  dimension "d56" = 50
  dimension "d57" = 50
  dimension "d58" = 50
  dimension "d59" = 50
  dimension "d60" = 50
  dimension "d61" = 5
  dimension "d62" = 5
  dimension "d63" = 55
  constraints: 8 end point, 5 centre point, 2 parallel, 1 horizontal, 1 midpoint, 1 perpendicular
  measures "d44" distance of L2.end L1.end
  measures "d45" distance of L1.end L0.end
  measures "d46" distance between parallel lines of L4 L5
  measures "d47" distance from line of L5 point (40, 85)
  measures "d50" distance between parallel lines of L6 L1
  measures "d51" diameter of A0
  measures "d52" diameter of A1
  measures "d53" diameter of A2
  measures "d54" diameter of A3
  measures "d55" distance of A3.centre A0.centre
  measures "d56" horizontal distance of A2.centre A0.centre
  measures "d57" distance of A2.centre A3.centre
  measures "d58" distance of A1.centre A2.centre
  measures "d59" distance of A1.centre A0.centre
  measures "d60" horizontal distance of A1.centre A3.centre
  measures "d61" distance from line of L0 A0.centre
  measures "d62" distance from line of L1 A3.centre
  measures "d63" diameter of A4
extrude "돌출6" cut sketch "스케치6" against normal blind 5 contours A0 | A1 | A2 | A3 | A4
